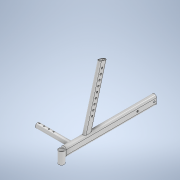
# Autodesk Inventor part: Liftarm
Saved by Autodesk Inventor 2022 (Build 260153000, 153)
## iProperties
Created: 2021-12-04
Part Number: Liftarm
Material: Generic
Document SubType Name: Modeling
Designer: Vedic
Density: 1 g/cm^3
Appearance: Default
Author: Vedic
Autodesk Inventor part; units mm, degrees
sketch "Sketch1" plane through (0, 0, 0) normal (0, 0, 1) x (1, 0, 0)
  line L0 (-12.7, -12.7) -> (-12.7, 12.7)
  arc A0 (12.7, 12.7) -> (-12.7, 12.7) centre (0, 12.7) ccw
  line L1 (12.7, 12.7) -> (12.7, -12.7)
  arc A1 (-12.7, -12.7) -> (12.7, -12.7) centre (0, -12.7) ccw
  line L2 (-10.16, 12.7) -> (-10.16, -12.7)
  arc A2 (-10.16, -12.7) -> (10.16, -12.7) centre (0, -12.7) ccw
  line L3 (10.16, -12.7) -> (10.16, 12.7)
  arc A3 (10.16, 12.7) -> (-10.16, 12.7) centre (0, 12.7) ccw
  point P0 (0, 0)
  dimension "d0" = 25.4
  dimension "d1" = 25.4
  dimension "d2" = 12.7
  dimension "d3" = 12.7
  dimension "d22" = 2.54
  constraints: 8 end point, 8 point on circle, 4 centre point, 4 tangent, 2 parallel, 1 vertical, 3 other
  measures "d0" distance between parallel lines of L1 L0
  measures "d1" distance of L0.start L0.end
  measures "d2" distance of A1.centre point (0, 0)
  measures "d3" distance from line of L0 point (0, 0)
  measures "d22" distance between parallel lines of L1 L3
ref_plane "Work Plane5" through (-12.7, -12.7, 63.5) normal (0, 0, -1) x (0, 1, 0)
ref_plane "Work Plane4" through (-12.7, -12.7, 0) normal (0, 0, -1) x (0, 1, 0)
sketch "Sketch5" plane through (-12.7, -12.7, 63.5) normal (0, 0, -1) x (0, 1, 0)
  line L0 (38.1, 50.8) -> (63.5, 50.8)
  arc A0 (38.1, 76.2) -> (38.1, 50.8) centre (38.1, 63.5) ccw
  line L1 (38.1, 76.2) -> (63.5, 76.2)
  arc A1 (63.5, 50.8) -> (63.5, 76.2) centre (63.5, 63.5) ccw
  line L2 (50.8, 50.8) -> (50.8, 76.2) construction
  line L3 (63.5, 63.5) -> (38.1, 63.5) construction
  line L4 (12.7, 12.7) -> (50.8, 12.7) construction
  line L5 (50.8, 12.7) -> (50.8, 63.5) construction
  line L6 (50.8, 63.5) -> (12.7, 63.5) construction
  line L7 (12.7, 63.5) -> (12.7, 12.7) construction
  line L8 (63.5, 73.66) -> (38.1, 73.66)
  arc A2 (38.1, 73.66) -> (38.1, 53.34) centre (38.1, 63.5) ccw
  line L9 (38.1, 53.34) -> (63.5, 53.34)
  arc A3 (63.5, 53.34) -> (63.5, 73.66) centre (63.5, 63.5) ccw
  dimension "d24" = 25.4
  dimension "d25" = 25.4
  dimension "d26" = 38.1
  dimension "d27" = 50.8
  dimension "d28" = 2.54
  constraints: 20 end point, 8 point on circle, 4 centre point, 4 parallel, 3 horizontal, 3 midpoint, 3 tangent, 1 perpendicular, 3 other
  measures "d24" distance of L1.start L1.end
  measures "d25" distance between parallel lines of L1 L0
  measures "d26" distance of L5.end L6.end
  measures "d27" distance of L4.end L5.end
  measures "d28" distance between parallel lines of L1 L8
loft "Loft3" add profiles "Sketch5", "Sketch1" contours A0 L1 A1 L0 | A3 L9 A2 L8 / L0 A0 L1 A1 | A3 L3 A2 L2
loft "Loft4" cut profiles "Sketch5", "Sketch1" contours A3 L9 A2 L8 / A3 L3 A2 L2
extrude "Extrusion1" add sketch "Sketch1" against normal blind 482.6
ref_plane "Work Plane6" through (0, 38.1, 63.5) normal (0, -1, 0) x (1, 0, 0)
sketch "Sketch6" plane through (0, 38.1, 63.5) normal (0, -1, 0) x (1, 0, 0)
  line L0 (0, -63.5) -> (50.8, 0)
  line L1 (40.64, 0) -> (60.96, 0) projected
  circle A0 centre (50.8, 0) radius 14.605
  dimension "d47" = 29.21
  constraints: 2 end point, 1 centre point, 1 coincident, 1 midpoint
  measures "d47" diameter of A0
extrude "Extrusion2" add sketch "Sketch6" along normal mid plane 69.85
sketch "Sketch8" plane through (50.8, 73.025, 63.5) normal (0, 1, 0) x (1, 0, 0)
  circle A0 centre (0, 0) radius 14.605 projected
  circle A1 centre (0, 0) radius 12.7
  point P0 (-50.8, 63.5)
  constraints: 1 centre point, 1 coincident
extrude "Extrusion4" cut sketch "Sketch8" against normal blind 8.89 contours A0 | A1
sketch "Sketch9" plane through (50.8, 64.135, 63.5) normal (0, 1, 0) x (1, 0, 0)
  circle A0 centre (0, 0) radius 14.605 projected
  circle A1 centre (0, 0) radius 11.43
  point P0 (-50.8, 63.5)
  point P1 (-7.1569, 12.7313)
  point P2 (-10.043, 10.604)
  dimension "d50" = 22.86
  constraints: 1 centre point, 1 coincident
  measures "d50" diameter of A1
extrude "Extrusion5" cut sketch "Sketch9" against normal blind 50.8 contours A1
sketch "Sketch10" plane through (50.8, 13.335, 63.5) normal (0, 1, 0) x (1, 0, 0)
  circle A0 centre (0, 0) radius 11.43 projected
  circle A1 centre (0, 0) radius 4.7625
  point P0 (-50.8, 63.5)
  dimension "d53" = 9.525
  constraints: 1 centre point, 1 coincident
  measures "d53" diameter of A1
hole "Hole1" at (50.8, 13.335, 63.5) direction (0, -1, 0) diameter 9.525 end through all
sketch "Sketch11" plane through (-12.7, -12.7, -482.6) normal (-1, 0, 0) x (0, 0, 1)
  circle A0 centre (431.8, 12.7) radius 12.7
  line L0 (482.6, 12.7) -> (431.8, 12.7)
  line L1 (431.8, 12.7) -> (431.8, 12.7)
  line L2 (431.8, 12.7) -> (482.6, 12.7)
  line L3 (482.6, 12.7) -> (482.6, 12.7)
  circle A1 centre (431.8, 12.7) radius 9.525
  dimension "d65" = 25.4
  dimension "d66" = 0
  dimension "d67" = 50.8
  dimension "d69" = 19.05
  constraints: 8 end point, 2 centre point, 2 equal length, 1 horizontal, 1 perpendicular
  measures "d65" diameter of A0
  measures "d66" distance of L2.end L0.start
  measures "d67" distance of L0.start L0.end
  measures "d69" diameter of A1
extrude "Extrusion6" add sketch "Sketch11" along normal blind 177.8
ref_plane "Work Plane7" through (-12.7, 12.7, 0) normal (0, 1, 0) x (-1, 0, 0)
sketch "Sketch12" plane through (-12.7, 12.7, 0) normal (0, 1, 0) x (-1, 0, 0)
  line L0 (177.8, -63.5) -> (177.8, -38.1) construction
  line L1 (0, -63.5) -> (177.8, -63.5) construction
  line L2 (177.8, -50.8) -> (0, -50.8) construction
  line L3 (0, -50.8) -> (0, -63.5) construction
  line L4 (0, -63.5) -> (177.8, -63.5) construction
  line L5 (177.8, -63.5) -> (177.8, -50.8) construction
  line L6 (0, 0) -> (0, -50.8) projected
  line L7 (177.8, -38.1) -> (0, -38.1) construction
  line L8 (0, -38.1) -> (0, -50.8) construction
  line L9 (0, -50.8) -> (177.8, -50.8) construction
  line L10 (177.8, -50.8) -> (177.8, -38.1) construction
  circle A0 centre (168.275, -50.8) radius 3.175
  circle A1 centre (142.875, -50.8) radius 3.175
  line L11 (177.8, -50.8) -> (168.275, -50.8) construction
  line L12 (168.275, -50.8) -> (142.875, -50.8) construction
  circle A2 centre (117.475, -50.8) radius 3.175
  circle A3 centre (92.075, -50.8) radius 3.175
  point P0 (-12.7, 0)
  dimension "d72" = 9.525
  dimension "d73" = 6.35
  dimension "d74" = 25.4
  dimension "d128" = 25.4
  dimension "d129" = 25.4
  constraints: 20 end point, 5 point on line, 4 centre point, 4 parallel, 3 equal radius, 2 collinear, 2 horizontal, 2 perpendicular, 1 midpoint
  measures "d72" distance of L2.start L11.end
  measures "d73" diameter of A0
  measures "d74" distance of L12.end L11.end
  measures "d128" distance of A2.centre L12.end
  measures "d129" distance of A3.centre A2.centre
extrude "Extrusion7" cut sketch "Sketch12" against normal through all
ref_plane "Work Plane8" through (-12.7, 22.225, 0) normal (0, 1, 0) x (-1, 0, 0)
sketch "Sketch13" plane through (-12.7, 22.225, 0) normal (0, 1, 0) x (-1, 0, 0)
  line L0 (-4.3053, -109.9947) -> (-4.3053, -135.3947)
  arc A0 (-21.0947, -135.3947) -> (-4.3053, -135.3947) centre (-12.7, -135.3947) ccw
  line L1 (-21.0947, -135.3947) -> (-21.0947, -109.9947)
  arc A1 (-4.3053, -109.9947) -> (-21.0947, -109.9947) centre (-12.7, -109.9947) ccw
  line L2 (-25.4, 0) -> (-25.4, -482.6) projected
  line L3 (0, -50.8) -> (0, -482.6) projected
  line L4 (-12.7, -101.6) -> (-12.7, -143.7894) construction
  line L5 (-6.604, 0) -> (-22.86, 0) construction
  line L6 (-18.5547, -109.9947) -> (-18.5547, -135.3947)
  arc A2 (-18.5547, -135.3947) -> (-6.8453, -135.3947) centre (-12.7, -135.3947) ccw
  line L7 (-6.8453, -135.3947) -> (-6.8453, -109.9947)
  arc A3 (-6.8453, -109.9947) -> (-18.5547, -109.9947) centre (-12.7, -109.9947) ccw
  dimension "d84" = 25.4
  dimension "d85" = 16.7894
  dimension "d86" = 4.3053
  dimension "d87" = 4.3053
  dimension "d88" = 101.6
  dimension "d96" = 2.54
  constraints: 10 end point, 10 point on circle, 4 centre point, 4 tangent, 2 vertical, 3 other
  measures "d84" distance of L1.start L1.end
  measures "d85" distance between parallel lines of L1 L0
  measures "d86" distance between parallel lines of L1 L2
  measures "d87" distance between parallel lines of L3 L0
  measures "d88" distance from line of L5 L4.start
  measures "d96" distance between parallel lines of L1 L6
extrude "Extrusion8" cut sketch "Sketch13" along normal blind 25.4 contours L0 A0 L1 A1 | A3 L7 A2 L6
ref_plane "Work Plane9" through (-12.7, 327.025, 0) normal (0, 1, 0) x (1, 0, 0)
sketch "Sketch14" plane through (-12.7, 327.025, 0) normal (0, 1, 0) x (1, 0, 0)
  line L0 (4.3053, 192.5447) -> (4.3053, 217.9447)
  arc A0 (21.0947, 217.9447) -> (4.3053, 217.9447) centre (12.7, 217.9447) ccw
  line L1 (21.0947, 217.9447) -> (21.0947, 192.5447)
  arc A1 (4.3053, 192.5447) -> (21.0947, 192.5447) centre (12.7, 192.5447) ccw
  line L2 (21.0947, 135.3947) -> (21.0947, 109.9947) projected
  line L3 (18.5547, 192.5447) -> (18.5547, 217.9447)
  arc A2 (18.5547, 217.9447) -> (6.8453, 217.9447) centre (12.7, 217.9447) ccw
  line L4 (6.8453, 217.9447) -> (6.8453, 192.5447)
  arc A3 (6.8453, 192.5447) -> (18.5547, 192.5447) centre (12.7, 192.5447) ccw
  point P0 (12.7, 0)
  dimension "d92" = 25.4
  dimension "d93" = 16.7894
  dimension "d94" = 0
  dimension "d95" = 82.55
  dimension "d97" = 2.54
  constraints: 8 end point, 8 point on circle, 4 centre point, 4 tangent, 2 parallel, 1 vertical, 3 other
  measures "d92" distance of L1.start L1.end
  measures "d93" distance between parallel lines of L0 L1
  measures "d94" distance between parallel lines of L1 L2
  measures "d95" distance of L1.start L2.start
  measures "d97" distance between parallel lines of L1 L3
loft "Loft5" add profiles "Sketch13", "Sketch14" contours L0 A0 L1 A1 | A3 L7 A2 L6 / L0 A0 L1 A1 | A3 L4 A2 L3
loft "Loft6" cut profiles "Sketch14", "Sketch13" contours A3 L4 A2 L3 / A3 L7 A2 L6
sketch "Sketch15" plane through (8.3947, 327.025, -192.5447) normal (1, 0, 0) x (0, 0, -1)
  line L0 (-8.3947, 0) -> (0, 0) projected
  line L1 (-8.3947, 0) -> (23.0905, -8.5273)
  line L2 (-57.1487, -304.7951) -> (25.4, 0) projected
  line L3 (-57.1487, -304.7951) -> (25.4, 0) projected
  line L4 (23.0905, -8.5273) -> (43.483, -14.0502)
  line L5 (43.483, -14.0502) -> (50.3622, 11.3498)
  line L6 (50.3622, 11.3498) -> (-23.1881, 31.2696)
  line L7 (-23.1881, 31.2696) -> (-30.0672, 5.8696)
  line L8 (-30.0672, 5.8696) -> (-8.3947, 0)
  point P0 (-192.5447, -327.025)
  dimension "d106" = 25.4
  dimension "d107" = 76.2
  constraints: 12 end point, 5 perpendicular, 1 collinear, 1 point on line
  measures "d106" vertical distance of L4.end L5.end
  measures "d107" distance of L5.end L6.end
extrude "Extrusion9" cut sketch "Sketch15" against normal through all
sketch "Sketch17" plane through (12.7, -12.7, -482.6) normal (1, 0, 0) x (0, 0, -1)
  line L0 (-482.6, 12.7) -> (0, 12.7) construction
  line L1 (0, 25.4) -> (0, 0) construction
  circle A0 centre (-101.6, 12.7) radius 4.7625
  circle A1 centre (-12.7, 12.7) radius 4.7625
  dimension "d121" = 9.525
  dimension "d122" = 9.525
  dimension "d123" = 12.7
  dimension "d124" = 101.6
  constraints: 2 centre point, 2 end point, 2 point on line, 1 midpoint
  measures "d121" diameter of A0
  measures "d122" diameter of A1
  measures "d123" distance of L0.end A1.centre
  measures "d124" distance of L0.end A0.centre
extrude "Extrusion11" cut sketch "Sketch17" against normal through all
sketch "Sketch18" plane through (8.3947, 22.2299, -109.996) normal (1, 0, 0) x (0, 0, -1)
  line L0 (0, 0) -> (25.3987, 0) construction
  line L1 (12.6993, 0) -> (93.8071, 299.4724) construction
  line L2 (105.6392, 296.2678) -> (81.975, 302.6769) construction
  circle A0 centre (85.5071, 268.8265) radius 4.7625
  circle A1 centre (78.8671, 244.3097) radius 4.7625
  circle A2 centre (72.2271, 219.793) radius 4.7625
  circle A3 centre (65.5871, 195.2762) radius 4.7625
  circle A4 centre (58.9471, 170.7595) radius 4.7625
  circle A5 centre (52.3071, 146.2428) radius 4.7625
  circle A6 centre (45.6671, 121.726) radius 4.7625
  circle A7 centre (39.0271, 97.2093) radius 4.7625
  circle A8 centre (32.3871, 72.6926) radius 4.7625
  point P0 (-109.996, -22.2299)
  dimension "d130" = 31.75
  dimension "d131" = 9.525
  dimension "d134" = 25.4
  constraints: 9 centre point, 2 end point, 2 midpoint, 1 point on line, 17 other
  measures "d130" distance from line of L2 A0.centre
  measures "d131" diameter of A0
  measures "d134" distance of A0.centre A1.centre
extrude "Extrusion12" cut sketch "Sketch18" against normal blind 25.4
equation "\"d2\" = 0.5 * d1"
equation "\"d3\" = 0.5 * d0"
equation "\"d24\" = d1"
equation "\"d25\" = d0"
equation "\"d28\" = d22"
equation "\"d128\" = d74"
equation "\"d129\" = d74"
equation "\"d86\" = d87"
equation "\"d92\" = d84"
equation "\"d93\" = d85"
equation "\"d97\" = d96"
equation "\"d121\" = d122"
body "Solid3"
